Autodesk Fusion 360 part; units mm, degrees
(part 2 of 2)
extrude "Extrude1" add sketch "Sketch3" along normal blind 1 contours L0 L1 L2 L3 | L4 L5 L6 L7 picked at (-42.727796, 61.16077) picked at (-42.685053, -7.617249)
extrude "Extrude2" cut sketch "Sketch2" along normal blind 1 contours L0 L1 L2 L3 A0 A1 A2 A3 | L4 L5 L6 L7 A4 A5 A6 A7 | L8 L9 L10 L11 A8 A9 A10 A11 | L12 L13 L14 L15 A12 A13 A14 A15 | L16 L17 L18 L19 A16 A17 A18 A19 | L20 L21 L22 L23 A20 A21 A22 A23 | L24 L25 L26 L27 A24 A25 A26 A27 | L28 L29 L30 L31 A28 A29 A30 A31 | L32 L33 L34 L35 A32 A33 A34 A35 | L36 L37 L38 L39 A36 A37 A38 A39 | L40 L41 L42 L43 A40 A41 A42 A43 | L44 L45 L46 L47 A44 A45 A46 A47 | L48 L49 L50 L51 A48 A49 A50 A51 | L52 L53 L54 L55 A52 A53 A54 A55 | L56 L57 L58 L59 A56 A57 A58 A59 | L60 L61 L62 L63 A60 A61 A62 A63 | L64 L65 L66 L67 A64 A65 A66 A67 | L68 L69 L70 L71 A68 A69 A70 A71 | L72 L73 L74 L75 A72 A73 A74 A75 | L76 L77 L78 L79 A76 A77 A78 A79 | L80 L81 L82 L83 A80 A81 A82 A83 | L84 L85 L86 L87 A84 A85 A86 A87 | L88 L89 L90 L91 A88 A89 A90 A91 | L92 L93 L94 L95 A92 A93 A94 A95 | L96 L97 L98 L99 A96 A97 A98 A99 | L100 L101 L102 L103 A100 A101 A102 A103 | L104 L105 L106 L107 A104 A105 A106 A107 | L108 L109 L110 L111 A108 A109 A110 A111 | L112 L113 L114 L115 A112 A113 A114 A115 | L116 L117 L118 L119 A116 A117 A118 A119 | L120 L121 L122 L123 A120 A121 A122 A123 | L124 L125 L126 L127 A124 A125 A126 A127 | L128 L129 L130 L131 A128 A129 A130 A131 | L132 L133 L134 L135 A132 A133 A134 A135 | L136 L137 L138 L139 A136 A137 A138 A139 | L140 L141 L142 L143 A140 A141 A142 A143 | L144 L145 L146 L147 A144 A145 A146 A147 | L148 L149 L150 L151 A148 A149 A150 A151 | L152 L153 L154 L155 A152 A153 A154 A155 | L156 L157 L158 L159 A156 A157 A158 A159 | L160 L161 L162 L163 A160 A161 A162 A163 | L164 L165 L166 L167 A164 A165 A166 A167 | L168 L169 L170 L171 A168 A169 A170 A171 | L172 L173 L174 L175 A172 A173 A174 A175 | L176 L177 L178 L179 A176 A177 A178 A179 | L180 L181 L182 L183 A180 A181 A182 A183 | L184 L185 L186 L187 A184 A185 A186 A187 | L188 L189 L190 L191 A188 A189 A190 A191 | L192 L193 L194 L195 A192 A193 A194 A195 | L196 L197 L198 L199 A196 A197 A198 A199 | L200 L201 L202 L203 A200 A201 A202 A203 | L204 L205 L206 L207 A204 A205 A206 A207 | L208 L209 L210 L211 A208 A209 A210 A211 | L212 L213 L214 L215 A212 A213 A214 A215 | L216 L217 L218 L219 A216 A217 A218 A219 | L220 L221 L222 L223 A220 A221 A222 A223 | L224 L225 L226 L227 A224 A225 A226 A227 | L228 L229 L230 L231 A228 A229 A230 A231 | L232 L233 L234 L235 A232 A233 A234 A235 | L236 L237 L238 L239 A236 A237 A238 A239 | L240 L241 L242 L243 A240 A241 A242 A243 | L244 L245 L246 L247 A244 A245 A246 A247 | L248 L249 L250 L251 A248 A249 A250 A251 | L252 L253 L254 L255 A252 A253 A254 A255 | L256 L257 L258 L259 A256 A257 A258 A259 | L260 L261 L262 L263 A260 A261 A262 A263 | L264 L265 L266 L267 A264 A265 A266 A267 | L268 L269 L270 L271 A268 A269 A270 A271 | L272 L273 L274 L275 A272 A273 A274 A275 | L276 L277 L278 L279 A276 A277 A278 A279 | L280 L281 L282 L283 A280 A281 A282 A283 picked at (-144.888053, 49.408751) picked at (-121.504719, 45.075418) picked at (-106.788053, 49.408751) picked at (-83.404719, 49.408751) picked at (-68.354719, 49.408751) picked at (-45.304719, 49.408751) picked at (-30.421386, 49.575418) picked at (-11.371386, 49.575418) picked at (7.678614, 49.575418) picked at (26.728614, 49.575418) picked at (45.945281, 49.408751) picked at (64.828614, 49.575418) picked at (83.878614, 49.575418) picked at (109.905697, 49.408751) picked at (136.432781, 49.408751) picked at (-140.125553, 30.358751) picked at (-116.146386, 25.858751) picked at (-92.596386, 26.025418) picked at (-73.546386, 26.025418) picked at (-54.829719, 26.025418) picked at (-39.946386, 30.525418) picked at (-20.896386, 30.525418) picked at (-1.846386, 25.858751) picked at (17.203614, 25.858751) picked at (36.420281, 30.358751) picked at (55.470281, 30.358751) picked at (78.686947, 25.858751) picked at (97.736947, 25.858751) picked at (115.001531, 26.025418) picked at (136.432781, 30.358751) picked at (-137.410969, 6.975418) picked at (-111.217219, 11.308751) picked at (-92.167219, 11.308751) picked at (-73.283886, 6.808751) picked at (-50.067219, 6.975418) picked at (-35.183886, 11.475418) picked at (-16.133886, 11.475418) picked at (2.916114, 6.808751) picked at (21.966114, 11.475418) picked at (41.016114, 11.475418) picked at (64.232781, 6.975418) picked at (83.282781, 6.975418) picked at (107.691114, 11.475418) picked at (96.753114, 9.975418) picked at (120.629114, 9.975418) picked at (136.432781, 6.975418) picked at (-130.696386, -12.074582) picked at (-146.134386, -9.074582) picked at (-122.258386, -9.074582) picked at (-106.621386, -12.241249) picked at (-83.238053, -7.574582) picked at (-64.021386, -12.074582) picked at (-45.304719, -12.074582) picked at (-26.088053, -7.574582) picked at (-7.038053, -7.574582) picked at (12.011947, -7.574582) picked at (26.728614, -7.574582) picked at (45.945281, -12.074582) picked at (64.828614, -7.574582) picked at (91.022364, -12.241249) picked at (117.382781, -12.074582) picked at (136.432781, -12.074582) picked at (-142.506803, -31.124582) picked at (-118.527636, -31.291249) picked at (-94.548469, -26.791249) picked at (-18.777636, -26.791249) picked at (48.159864, -26.624582) picked at (76.139031, -26.791249) picked at (98.166114, -31.291249) picked at (117.382781, -26.791249) picked at (136.432781, -26.791249)
sketch "Sketch4" plane through (0, 0, 0) normal (0, 0, 1) x (1, 0, 0)
  line L0 (159.404281, 64.141947) -> (174.404281, 64.141947)
  line L1 (174.404281, 64.141947) -> (174.404281, 49.141947)
  line L2 (174.404281, 49.141947) -> (159.404281, 49.141947)
  line L3 (159.404281, 49.141947) -> (159.404281, 64.141947)
  line L4 (186.804281, 64.142084) -> (186.804281, -45.996916)
  line L5 (181.804281, 59.142084) -> (181.804281, -40.996916)
  dimension "d18" = 15
  dimension "d19" = 15
  dimension "d21" = 7.4
  constraint horizontal L0
  constraint vertical L1
  constraint horizontal L2
  constraint vertical L3
  measures "d21" distance of L1 L5
extrude "Extrude3" cut sketch "Sketch4" along normal blind 1 contours L0 L1 L2 L3 picked at (164.404281, 59.141947)
other "Base Mesh Feature2"
other "MeshRepair1"
other "Modify3"
other "Base Mesh Feature3"
other "Modify4"
other "Modify5"
other "CopyPasteMeshes1"
other "Modify6"
move_body "Move1" bodies 1 to x (1, 0, 0) y (0, 1, 0) z (0, 0, 1) at (0, 0, 6)
other "Modify7"
other "Modify8"
sketch "Sketch6" plane through (0, 0, 0) normal (0, 0, 1) x (1, 0, 0)
  line L0 (-80.000001, -20) -> (-63.000001, -20)
  line L1 (-63.000001, -20) -> (-63.000001, -40.000001)
  line L2 (-63.000001, -40.000001) -> (-80.000001, -40.000001)
  line L3 (-80.000001, -40.000001) -> (-80.000001, -20)
  line L4 (19, -20) -> (36.000001, -20)
  line L5 (36.000001, -20) -> (36.000001, -40.000001)
  line L6 (36.000001, -40.000001) -> (19, -40.000001)
  line L7 (19, -40.000001) -> (19, -20)
  line L8 (-78.000001, -40.000001) -> (-78.000001, -21)
  line L9 (21, -40.000001) -> (21, -21)
  line L10 (-28.110969, -22.457916) -> (-28.110969, -35.457916)
  line L11 (-14.110969, -22.457916) -> (-14.110969, -35.457916)
  point P0 (21, -40.000001)
  dimension "d26" = 17
  dimension "d27" = 17
  dimension "d28" = 20
  dimension "d29" = 20
  dimension "d30" = 2
  dimension "d31" = 2
  dimension "d32" = 34.889032
  dimension "d33" = 33.11097
  constraint horizontal L0
  constraint vertical L1
  constraint horizontal L2
  constraint vertical L3
  constraint horizontal L4
  constraint vertical L5
  constraint horizontal L6
  constraint vertical L7
  measures "d26" distance of L1 L3
  measures "d27" distance of L5 L7
  measures "d28" distance of L0 L2
  measures "d30" distance of L3 L8
  measures "d31" distance of L7 L9
  measures "d32" distance of L1 L10
  measures "d33" distance of L7 L11
extrude "Extrude5" cut sketch "Sketch6" along normal blind 7 contours L0 L1 L2 L3 | L4 L5 L6 L7 picked at (-73.666668, -26.666667) picked at (25.333334, -26.666667)
fillet "Fillet1" radius 1.25 1 edges at (186.804281, 64.142084, 6.5)
fillet "Fillet2" radius 1.25 1 edges at (186.804281, -45.996916, 6.5)
fillet "Fillet3" radius 1.25 1 edges at (-159.929719, -45.996916, 6.5)
fillet "Fillet4" radius 1.25 1 edges at (-159.929719, 64.142084, 6.5)
fillet "Fillet5" radius 0.75 1 edges at (182.90579, 62.184507, 7)
fillet "Fillet6" radius 0.75 1 edges at (182.90579, -42.954493, 7)
fillet "Fillet7" radius 0.75 1 edges at (-158.82821, -42.954493, 7)
fillet "Fillet8" radius 0.75 1 edges at (-158.82821, 62.184507, 7)
